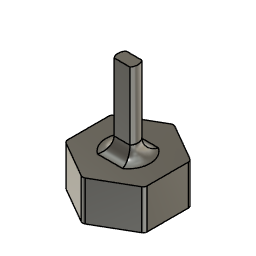
motor+manual (Autodesk Fusion 360 design; units mm, degrees)
Autodesk Fusion 360 part; units mm, degrees
sketch "Boceto1" plane through (0, 0, 0) normal (0, 0, 1) x (1, 0, 0)
  circle A0 centre (0, 0) radius 2.5
  line L0 (9.5, 6.0622) -> (0.5, 11.2583)
  line L1 (-0.5, 11.2583) -> (-9.5, 6.0622)
  line L2 (-10, 5.1962) -> (-10, -5.1962)
  line L3 (-9.5, -6.0622) -> (-0.5, -11.2583)
  line L4 (0.5, -11.2583) -> (9.5, -6.0622)
  line L5 (10, -5.1962) -> (10, 5.1962)
  line L6 (-2, 1.5) -> (2, 1.5)
  line L7 (-2, -1.5) -> (2, -1.5)
  arc A1 (-9.5, 6.0622) -> (-10, 5.1962) centre (-9, 5.1962) ccw
  arc A2 (0.5, 11.2583) -> (-0.5, 11.2583) centre (0, 10.3923) ccw
  arc A3 (10, 5.1962) -> (9.5, 6.0622) centre (9, 5.1962) ccw
  arc A4 (9.5, -6.0622) -> (10, -5.1962) centre (9, -5.1962) ccw
  arc A5 (-0.5, -11.2583) -> (0.5, -11.2583) centre (0, -10.3923) ccw
  arc A6 (-10, -5.1962) -> (-9.5, -6.0622) centre (-9, -5.1962) ccw
  dimension "d1" = 3
  dimension "d2" = 1.5
  dimension "d3" = 5
  dimension "d4" = 20
  dimension "d11" = 1
  dimension "d12" = 10
  dimension "d13" = 10
  dimension "d14" = 10
  constraint coincident A0.centre origin
  constraint coincident A0 L6.start
  constraint coincident A0 L6.end
  constraint horizontal L6
  constraint coincident A0 L7.start
  constraint coincident A0 L7.end
  constraint horizontal L7
  constraint vertical L5
  constraint tangent L1 A1
  constraint tangent L2 A1
  constraint tangent L0 A2
  constraint tangent L1 A2
  constraint equal A1 A2
  constraint tangent L0 A3
  constraint tangent L5 A3
  constraint equal A1 A3
  constraint tangent L4 A4
  constraint tangent L5 A4
  constraint equal A1 A4
  constraint tangent L3 A5
  constraint tangent L4 A5
  constraint equal A1 A5
  constraint tangent L2 A6
  constraint tangent L3 A6
  constraint equal A1 A6
  constraint equal L3 L4
  constraint equal L2 L3
  constraint equal L1 L2
  constraint equal L0 L1
  constraint equal L0 L5
  constraint horizontal A4.centre A6.centre
  measures "d1" distance of L6 L7
  measures "d2" distance of A0.centre L6
  measures "d3" diameter of A0
  measures "d4" distance of L2 L5
  measures "d11" radius of A1
  measures "d12" distance of A0.centre L5
  measures "d13" distance of A0.centre L3
  measures "d14" distance of A0.centre L1
extrude "Extruir1" add sketch "Boceto1" along normal blind 20 contours A0 L6 L7
extrude "Extruir2" add sketch "Boceto1" against normal blind 10 contours A0 L6 L7 | A0 L6 | A0 L7 | L0 L1 L2 L3 L4 L5 A1 A2 A3 A4 A5 A6
fillet "Empalme1" radius 3 4 edges at (2.5, 0, 0) (0, -1.5, 0) (0, 1.5, 0) (-2.5, 0, 0)
equation "d2 = d1 / 2"
equation "d12 = d4 / 2"
